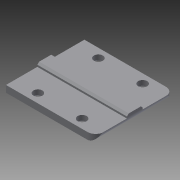
# Autodesk Inventor part: RearCarriageSupport
Saved by Autodesk Inventor 2015 (Build 190159000, 159)
## iProperties
Created: 2015-05-12
Part Number: RearCarriageSupport
Material: Generic
Document SubType Name: Modeling
Designer: Quinn
Density: 1 g/cm^3
Appearance: Default
Author: Quinn
Autodesk Inventor part; units mm, degrees
ref_plane "YZ Plane" through (0, 0, 0) normal (1, 0, 0) x (0, 1, 0)
ref_plane "XZ Plane" through (0, 0, 0) normal (0, 1, 0) x (-1, 0, 0)
ref_plane "XY Plane" through (0, 0, 0) normal (0, 0, 1) x (1, 0, 0)
sketch "Sketch2" plane through (0, 0, 0) normal (0, 1, 0) x (-1, 0, 0)
  line L0 (20, 17.5) -> (-20, 17.5)
  line L1 (-20, 17.5) -> (-20, -17.5)
  line L2 (-20, -17.5) -> (20, -17.5)
  line L3 (20, -17.5) -> (20, 17.5)
  point P0 (0, 0)
  point P1 (20, 0)
  point P2 (0, -17.5)
  dimension "d0" = 40
  dimension "d1" = 35
  constraints: 8 end point, 2 midpoint, 2 parallel, 1 horizontal, 1 horizontal alignment, 1 perpendicular, 1 vertical alignment
  measures "d0" distance of L2.end L1.end
  measures "d1" distance of L1.end L0.end
extrude "Extrusion1" add sketch "Sketch2" along normal blind 3
sketch "Sketch3" plane through (0, 3, 0) normal (0, 1, 0) x (1, 0, 0)
  line L0 (-20, -17.5) -> (20, -17.5) projected
  line L1 (20, -17.5) -> (20, 17.5) projected
  line L2 (20, 17.5) -> (-20, 17.5) projected
  line L3 (-20, 17.5) -> (-20, -17.5) projected
  line L4 (-20, 0) -> (20, 0)
  line L5 (0, 0) -> (-9.75, 0)
  line L6 (-9.75, 0) -> (-9.75, 17.5)
  line L7 (0, 0) -> (9.75, 0)
  line L8 (9.75, 0) -> (9.75, 17.5)
  line L9 (0, 0) -> (0, 13.5)
  line L10 (0, 13.5) -> (-20, 13.5)
  line L11 (0, 13.5) -> (20, 13.5)
  circle A0 centre (10, 13.5) radius 2
  circle A1 centre (-9.75, 13.5) radius 2
  circle A2 centre (10, -13.5) radius 2
  circle A3 centre (-9.75, -13.5) radius 2
  dimension "d4" = 9.75
  dimension "d5" = 9.75
  dimension "d6" = 13.5
  dimension "d7" = 4
  dimension "d8" = 4
  constraints: 16 end point, 9 point on line, 4 centre point, 4 perpendicular, 3 midpoint, 2 symmetric about line, 2 other
  measures "d4" distance of L5.start L5.end
  measures "d5" distance of L5.start L7.end
  measures "d6" distance of L5.start L9.end
  measures "d7" diameter of A0
  measures "d8" diameter of A1
extrude "Extrusion2" cut sketch "Sketch3" against normal through all contours A1 L6 L10 | L10 L6 A1 | L6 L10 A1 | A0 L8 L11 | L11 L8 A0 | A0 L11 L8 | L6 A1 L10 | L11 A0 L8 | A2 | A3
sketch "Sketch4" plane through (0, 3, 0) normal (0, 1, 0) x (1, 0, 0)
  circle A0 centre (10, -13.5) radius 2 projected
  circle A1 centre (-9.75, 13.5) radius 2 projected
  circle A2 centre (10, 13.5) radius 2 projected
  circle A3 centre (-9.75, -13.5) radius 2 projected
  line L0 (-20, -17.5) -> (20, -17.5) projected
  line L1 (20, -17.5) -> (20, 17.5) projected
  line L2 (20, 17.5) -> (-20, 17.5) projected
  line L3 (-20, 17.5) -> (-20, -17.5) projected
  line L4 (20, -3.5) -> (-20, -3.5)
  line L5 (-20, -3.5) -> (-20, 3.5)
  line L6 (-20, 3.5) -> (20, 3.5)
  line L7 (20, 3.5) -> (20, -3.5)
  line L8 (20, -3.5) -> (-20, 3.5) construction
  line L9 (-20, -3.5) -> (20, 3.5) construction
  point P0 (0, 0)
  dimension "d11" = 7
  constraints: 12 end point, 2 midpoint, 2 parallel, 1 horizontal, 1 perpendicular, 1 point on line
  measures "d11" distance of L4.end L5.end
extrude "Extrusion3" add sketch "Sketch4" along normal blind 1.6 contours L3 L6 L1 L4
fillet "Fillet1" radius 3.5875 3 edges at (20, 1.5, 17.5) (20, 1.5, -17.5) (20, 0, 0)
sketch "Sketch5" plane through (0, 0, 0) normal (0, -1, 0) x (1, 0, 0)
  circle A0 centre (-9.75, 13.5) radius 2 projected
  circle A1 centre (10, -13.5) radius 2 projected
  circle A2 centre (-9.75, -13.5) radius 2 projected
  circle A3 centre (10, 13.5) radius 2 projected
  line L0 (16.4125, 17.5) -> (16.4125, -17.5) projected
  line L1 (-20, 17.5) -> (16.4125, 17.5) projected
  line L2 (-20, -17.5) -> (-20, 17.5) projected
  line L3 (16.4125, -17.5) -> (-20, -17.5) projected
  circle A4 centre (-9.75, 13.5) radius 3
  circle A5 centre (10, 13.5) radius 3
  circle A6 centre (10, -13.5) radius 3
  circle A7 centre (-9.75, -13.5) radius 3
  point P0 (0, 0)
  dimension "d15" = 1
  dimension "d16" = 1
  dimension "d17" = 1
  dimension "d18" = 1
  constraints: 4 centre point
  measures "d15" radial gap between concentric circles of A0 A4
  measures "d16" radial gap between concentric circles of A3 A5
  measures "d17" radial gap between concentric circles of A1 A6
  measures "d18" radial gap between concentric circles of A2 A7
chamfer "Chamfer1" distance 0.8 angle 45 4 edges at (-11.75, 0, -13.5) (-11.75, 0, 13.5) (8, 0, 13.5) (8, 0, -13.5)
chamfer "Chamfer2" distance 0.8 angle 45 2 edges at (0, 4.6, 3.5) (0, 4.6, -3.5)
body "Solid1"
